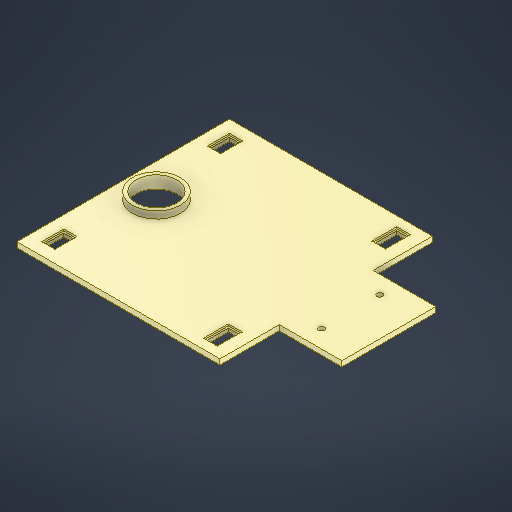
# Autodesk Inventor part: Base V.2
Saved by Autodesk Inventor 2026.2 (Build 302298010, 298A)
## iProperties
Created: 2026-05-06
Part Number: Base V.2
Material: Genérico
Document SubType Name: Modeling
Designer: migue
Density: 1 g/cm^3
Appearance: Nilón 6
Author: migue
Autodesk Inventor part; units mm, degrees
ref_plane "YZ Plane" through (0, 0, 0) normal (1, 0, 0) x (0, 1, 0)
ref_plane "XZ Plane" through (0, 0, 0) normal (0, 1, 0) x (-1, 0, 0)
ref_plane "XY Plane" through (0, 0, 0) normal (0, 0, 1) x (1, 0, 0)
sketch "Boceto1" plane through (0, 0, 0) normal (0, 1, 0) x (-1, 0, 0)
  line L0 (25.35, 26.5) -> (0, 26.5)
  line L1 (0, 26.5) -> (0, -26.5)
  line L2 (0, -26.5) -> (25.35, -26.5)
  line L3 (-8.9327, 0) -> (109.0416, 0) construction
  line L4 (25.35, 60) -> (150, 60)
  line L5 (150, 60) -> (150, -60)
  line L6 (150, -60) -> (25.35, -60)
  line L7 (25.35, -60) -> (25.35, -26.5)
  line L8 (25.35, 26.5) -> (25.35, 60)
  circle A0 centre (21.45, 16.5) radius 1.65
  circle A1 centre (21.45, -16.5) radius 1.65
  point P0 (0, 0)
  point P1 (0, 0)
  dimension "d1" = 53
  dimension "d2" = 120
  dimension "d3" = 124.65
  dimension "d4" = 25.35
  dimension "d6" = 33.5
  dimension "d8" = 3.3
  dimension "d9" = 16.5
  dimension "d10" = 3.9
  constraints: 18 end point, 5 parallel, 3 horizontal, 2 centre point, 2 perpendicular, 1 coincident, 1 midpoint, 1 symmetric about line, 1 other
  measures "d1" distance of L1.end L0.end
  measures "d2" distance of L4.end L5.end
  measures "d3" distance of L5.end L6.end
  measures "d4" distance of L1.end L2.end
  measures "d6" distance between parallel lines of L0 L4
  measures "d8" diameter of A0
  measures "d9" distance from line of L3 A0.centre
  measures "d10" distance from line of A0.centre L8
extrude "Extrusión1" add sketch "Boceto1" along normal blind 3
sketch "Boceto2" plane through (0, 3, 0) normal (0, 1, 0) x (1, 0, 0)
  line L0 (-150, 60) -> (-150, -60) projected
  line L1 (-25.35, 60) -> (-150, 60) projected
  line L2 (-150, -60) -> (-25.35, -60)
  line L3 (-25.35, -60) -> (-25.35, 60)
  line L4 (-25.35, 60) -> (-150, 60)
  line L5 (-150, 60) -> (-150, -60)
  line L6 (-30.35, -55) -> (-145, -55)
  line L7 (-145, -55) -> (-145, 55)
  line L8 (-145, 55) -> (-30.35, 55)
  line L9 (-30.35, 55) -> (-30.35, -55)
  circle A0 centre (-131.25, 0) radius 11.465
  circle A1 centre (-131.25, 0) radius 13.55
  point P0 (0, 0)
  dimension "d13" = 5
  dimension "d14" = 22.93
  dimension "d15" = 13.75
  dimension "d16" = 27.1
  constraints: 16 end point, 4 parallel, 2 centre point, 2 perpendicular, 1 coincident, 1 horizontal, 3 other
  measures "d13" distance between parallel lines of L2 L6
  measures "d14" diameter of A0
  measures "d15" distance from line of A0.centre L7
  measures "d16" diameter of A1
extrude "Extrusión2" cut sketch "Boceto2" against normal through all contours A0
extrude "Extrusión3" add sketch "Boceto2" along normal blind 4 contours A1
sketch "Boceto3" plane through (0, 3, 0) normal (0, 1, 0) x (1, 0, 0)
  line L0 (-25.35, 26.5) -> (-25.35, 60) projected
  line L1 (-25.35, 60) -> (-35.35, 60)
  line L2 (-35.35, 60) -> (-35.35, 26.5)
  line L3 (-35.35, 26.5) -> (-25.35, 26.5)
  line L4 (-25.35, 26.5) -> (-25.35, 60)
  line L5 (-25.35, -60) -> (-25.35, -26.5) projected
  line L6 (-25.35, -60) -> (-35.35, -60)
  line L7 (-35.35, -60) -> (-35.35, -26.5)
  line L8 (-35.35, -26.5) -> (-25.35, -26.5)
  line L9 (-25.35, -26.5) -> (-25.35, -60)
  point P0 (-150, 60)
  dimension "d46" = 10
  dimension "d47" = 10
  dimension "d48" = 33.5
  dimension "d49" = 33.5
  constraints: 16 end point, 4 parallel, 2 horizontal, 2 perpendicular
  measures "d46" distance of L3.end L2.end
  measures "d47" distance of L7.end L8.end
  measures "d48" distance of L6.end L7.end
  measures "d49" distance of L1.end L2.end
extrude "Extrusión7" cut sketch "Boceto3" against normal through all
sketch "Boceto4" plane through (0, 3, 0) normal (0, 1, 0) x (1, 0, 0)
  line L0 (-143, 53) -> (-135.55, 53)
  line L1 (-135.55, 53) -> (-135.55, 40.55)
  line L2 (-135.55, 40.55) -> (-143, 40.55)
  line L3 (-143, 40.55) -> (-143, 53)
  line L4 (-136.55, 52) -> (-142, 52)
  line L5 (-142, 52) -> (-142, 41.55)
  line L6 (-142, 41.55) -> (-136.55, 41.55)
  line L7 (-136.55, 41.55) -> (-136.55, 52)
  line L8 (-50.1, 54.55) -> (-42.35, 54.55)
  line L9 (-42.35, 54.55) -> (-42.35, 40.55)
  line L10 (-42.35, 40.55) -> (-50.1, 40.55)
  line L11 (-50.1, 40.55) -> (-50.1, 54.55)
  line L12 (-43.35, 53.55) -> (-49.1, 53.55)
  line L13 (-49.1, 53.55) -> (-49.1, 41.55)
  line L14 (-49.1, 41.55) -> (-43.35, 41.55)
  line L15 (-43.35, 41.55) -> (-43.35, 53.55)
  line L16 (-35.35, 60) -> (-150, 60) construction
  line L17 (-35.35, -26.5) -> (-35.35, -60) construction
  line L18 (-150, 60) -> (-35.35, 60) construction
  line L19 (-35.35, 60) -> (-35.35, -60) construction
  line L20 (-35.35, -60) -> (-150, -60) construction
  line L21 (-150, -60) -> (-150, 60) construction
  line L22 (-147, 57) -> (-38.35, 57) construction
  line L23 (-38.35, 57) -> (-38.35, -57) construction
  line L24 (-38.35, -57) -> (-147, -57) construction
  line L25 (-147, -57) -> (-147, 57) construction
  line L26 (-150, 0) -> (0, 0) construction
  line L27 (-50.1, -40.55) -> (-50.1, -54.55)
  line L28 (-136.55, -41.55) -> (-136.55, -52)
  line L29 (-135.55, -53) -> (-135.55, -40.55)
  line L30 (-136.55, -52) -> (-142, -52)
  line L31 (-142, -52) -> (-142, -41.55)
  line L32 (-142, -41.55) -> (-136.55, -41.55)
  line L33 (-143, -53) -> (-135.55, -53)
  line L34 (-135.55, -40.55) -> (-143, -40.55)
  line L35 (-143, -40.55) -> (-143, -53)
  line L36 (-42.35, -40.55) -> (-50.1, -40.55)
  line L37 (-42.35, -54.55) -> (-42.35, -40.55)
  line L38 (-50.1, -54.55) -> (-42.35, -54.55)
  line L39 (-43.35, -53.55) -> (-49.1, -53.55)
  line L40 (-49.1, -53.55) -> (-49.1, -41.55)
  line L41 (-49.1, -41.55) -> (-43.35, -41.55)
  line L42 (-43.35, -41.55) -> (-43.35, -53.55)
  point P0 (-46.225, 40.55)
  point P1 (-139.275, 40.55)
  point P2 (-46.225, -40.55)
  point P3 (-139.275, -40.55)
  dimension "d52" = 7.45
  dimension "d53" = 12.45
  dimension "d54" = 1
  dimension "d55" = 14
  dimension "d56" = 7.75
  dimension "d57" = 1
  dimension "d59" = 3
  dimension "d60" = 4
  dimension "d61" = 4
  dimension "d62" = 4
  constraints: 82 end point, 18 symmetric about line, 12 parallel, 6 perpendicular, 4 horizontal, 3 midpoint, 1 horizontal alignment, 9 other
  measures "d52" distance of L1.end L2.end
  measures "d53" distance of L1.start L1.end
  measures "d54" distance between parallel lines of L0 L4
  measures "d55" distance of L9.start L10.start
  measures "d56" distance of L10.start L11.start
  measures "d57" distance between parallel lines of L8 L12
  measures "d59" distance between parallel lines of L21 L25
  measures "d60" distance between parallel lines of L22 L0
  measures "d61" distance between parallel lines of L3 L25
  measures "d62" distance between parallel lines of L23 L9
extrude "Extrusión8" cut sketch "Boceto4" against normal blind 1
extrude "Extrusión9" cut sketch "Boceto4" against normal through all contours L7 L6 L5 L4 | L15 L14 L13 L12 | L28 L30 L31 L32 | L39 L40 L41 L42
